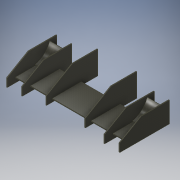
# Autodesk Inventor part: F-wing
Saved by Autodesk Inventor 2018.1 (Build 221171000, 171)
## iProperties
Created: 2017-10-11
Part Number: F-wing
Material: PAEK 樹脂
Document SubType Name: Modeling
Designer: kuwano
Density: 1.32 g/cm^3
Appearance: カーボンファイバー 1
Author: kuwano
Autodesk Inventor part; units mm, degrees
sketch "スケッチ1" plane through (0, 0, 0) normal (1, 0, 0) x (0, 1, 0)
  line L0 (10, 175) -> (0, 175)
  line L1 (0, 175) -> (0, -175)
  line L2 (0, -175) -> (10, -175)
  line L3 (10, -175) -> (10, 175)
  point P0 (0, 0)
  dimension "d0" = 350
  dimension "d1" = 10
  constraints: 8 end point, 2 midpoint, 2 parallel, 1 horizontal, 1 perpendicular
  measures "d0" distance of L0.end L1.end
  measures "d1" distance of L1.end L2.end
extrude "押し出し1" add sketch "スケッチ1" along normal mid plane 1350
sketch "スケッチ2" plane through (675, 0, 0) normal (1, 0, 0) x (0, 0, -1)
  line L0 (-15.1924, 200) -> (-275, 50)
  line L1 (-275, 50) -> (-275, -50)
  line L2 (-275, -50) -> (325, -50)
  line L3 (325, -50) -> (325, 200)
  line L4 (-175, 0) -> (175, 0) projected
  line L5 (-175, 10) -> (-175, 0) projected
  line L6 (175, 0) -> (175, 10) projected
  line L7 (175, 10) -> (-175, 10) projected
  line L8 (-15.1924, 200) -> (325, 200)
  point P0 (0, 0)
  dimension "d4" = 50
  dimension "d5" = 30
  dimension "d6" = 250
  dimension "d7" = 600
  dimension "d8" = 100
  dimension "d9" = 100
  constraints: 10 end point, 3 parallel, 1 horizontal
  measures "d4" distance between parallel lines of L2 L4
  measures "d5" angle of L7 L0
  measures "d6" distance of L2.end L3.end
  measures "d7" distance of L1.end L2.end
  measures "d8" distance between parallel lines of L5 L1
  measures "d9" distance of L0.end L1.end
extrude "押し出し3" add sketch "スケッチ2" along normal blind 10 contours L8 L3 L2 L1 L0 | L5 L7 L6 L4
ref_plane "作業平面1" through (230, 0, 0) normal (1, 0, 0) x (0, 1, 0)
ref_plane "作業平面2" through (589, 0, 0) normal (-1, 0, 0) x (0, 0, 1)
ref_plane "作業平面3" through (230, 0, 0) normal (1, 0, 0) x (0, 1, 0)
mirror "ミラー3" about plane through (589, 0, 0) normal (-1, 0, 0) of "押し出し3"
sketch "スケッチ4" plane through (230, 0, 0) normal (1, 0, 0) x (0, 1, 0)
  line L0 (70, 245) -> (-30, 245)
  line L1 (-30, 245) -> (-30, -375)
  line L2 (-30, -375) -> (250, -375)
  line L3 (250, -375) -> (250, -66.7691)
  line L4 (250, -66.7691) -> (70, 245)
  line L5 (0, -505) -> (0, 405) projected
  line L6 (50, 275) -> (-50, 275) projected
  line L7 (-50, 275) -> (-50, -325) projected
  line L8 (-50, -325) -> (200, -325) projected
  line L9 (200, -325) -> (200, 15.1924) projected
  point P0 (0, 0)
  dimension "d26" = 30
  dimension "d27" = 20
  dimension "d28" = 50
  dimension "d29" = 30
  dimension "d30" = 100
  dimension "d44" = 50
  constraints: 10 end point, 2 parallel, 1 horizontal, 1 perpendicular
  measures "d26" distance between parallel lines of L6 L0
  measures "d27" distance between parallel lines of L7 L1
  measures "d28" distance between parallel lines of L2 L8
  measures "d29" angle of L1 L4
  measures "d30" distance of L0.start L0.end
  measures "d44" distance between parallel lines of L9 L3
extrude "押し出し5" add sketch "スケッチ4" along normal blind 10 contours L4 L3 L2 L5 L0 | L5 L8 L1 L0 | L5 L2 L1 L8
sketch "スケッチ5" plane through (675, 0, 0) normal (-1, 0, 0) x (0, 0, 1)
  arc A0 (-243.2616, 197.5471) -> (-45, 20) centre (-11.1877, 257.2271) ccw
  line L0 (175, 10) -> (-175, 10) projected
  line L1 (-175, 10) -> (-175, 0) projected
  line L2 (-175, 10) -> (-243.2616, 197.5471)
  arc A1 (-243.2616, 197.5471) -> (-45, 20) centre (-61.7359, 200.7814) ccw
  point P0 (0, 0)
  dimension "d36" = 10
  dimension "d37" = 130
  dimension "d42" = 110
  constraints: 4 point on circle, 2 centre point, 2 end point
  measures "d36" distance from line of A0.end L0
  measures "d37" distance from line of A0.end L1
  measures "d42" angle of L0 L2
extrude "押し出し6" add sketch "スケッチ5" along normal up to next contours A0 L2 A1 | A0 A1 L2
fillet "フィレット1" radius 2 2 edges at (589, 197.5471, -243.2616) (589, 20, -45)
mirror "ミラー6" about plane through (0, 0, 0) normal (1, 0, 0) of "押し出し5", "押し出し3", "ミラー3", "押し出し6", "フィレット1"
